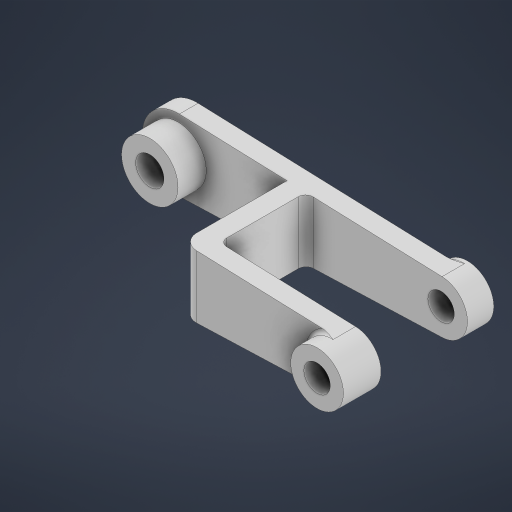
# Autodesk Inventor part: Part1
Saved by Autodesk Inventor 2023 (Build 270158000, 158)
## iProperties
Created: 2022-11-27
Part Number: Part1
Material: Generic
Document SubType Name: Modeling
Designer: iusti
Density: 1 g/cm^3
Appearance: Default
Author: iusti
Autodesk Inventor part; units mm, degrees
ref_plane "YZ Plane" through (0, 0, 0) normal (1, 0, 0) x (0, 1, 0)
ref_plane "XZ Plane" through (0, 0, 0) normal (0, 1, 0) x (-1, 0, 0)
sketch "Sketch1" plane through (0, 0, 0) normal (0, 0, 1) x (1, 0, 0)
  circle A0 centre (0, 0) radius 19
  circle A1 centre (140, 0) radius 14
  line L0 (0.678571, 18.987879) -> (140.5, 13.991069)
  line L1 (0.678571, -18.987879) -> (140.5, -13.991069)
  dimension "d0" = 38
  dimension "d1" = 28
  dimension "d2" = 140
  constraints: 4 end point, 4 point on circle, 4 tangent, 2 centre point, 1 coincident, 1 horizontal alignment
  measures "d0" diameter of A0
  measures "d1" diameter of A1
  measures "d2" distance of A1.centre point (0, 0)
extrude "Extrusion1" add sketch "Sketch1" along normal blind 10
ref_plane "Work Plane1" through (0, 0, 56) normal (0, 0, 1) x (1, 0, 0)
sketch "Sketch2" plane through (0, 0, 56) normal (0, 0, 1) x (1, 0, 0)
  line L0 (0.678571, -18.987879) -> (140.5, -13.991069) construction
  arc A0 (140.5, -13.991069) -> (140.5, 13.991069) centre (140, 0) ccw
  line L1 (140.5, 13.991069) -> (0.678571, 18.987879) construction
  arc A1 (0.678571, 18.987879) -> (0.678571, -18.987879) centre (0, 0) ccw construction
  line L2 (58, 16.939378) -> (58, -16.939378)
  line L3 (58, 16.939378) -> (140.5, 13.991069)
  line L4 (58, -16.939378) -> (140.5, -13.991069)
  arc A2 (140.5, -13.991069) -> (140.5, 13.991069) centre (140, 0) ccw
  dimension "d6" = 82
  constraints: 6 end point, 2 collinear, 2 point on circle, 2 point on line, 1 centre point, 1 coincident, 1 vertical
  measures "d6" distance from line of A0.centre L2
extrude "Extrusion2" add sketch "Sketch2" along normal blind 10
sketch "Sketch4" plane through (0, 0, 56) normal (0, 0, -1) x (-1, 0, 0)
  line L0 (-58, -16.939378) -> (-140.5, -13.991069)
  line L1 (-58, 16.939378) -> (-58, -16.939378)
  line L2 (-140.5, 13.991069) -> (-58, 16.939378)
  line L3 (-140.5, 13.991069) -> (-58, 16.939378)
  line L4 (-68, 16.582007) -> (-68, -16.582007)
  point P0 (0, 0)
  dimension "d10" = 10
  constraints: 2 end point, 2 point on line, 1 vertical
  measures "d10" distance between parallel lines of L1 L4
extrude "Extrusion3" add sketch "Sketch4" along normal up to next
fillet "Fillet1" radius 4 2 edges at (68, 0, 10) (68, 0, 56)
fillet "Fillet2" radius 8 1 edges at (58, 0, 66)
sketch "Sketch5" plane through (0, 0, 66) normal (0, 0, 1) x (1, 0, 0)
  arc A0 (140.5, -13.991069) -> (140.5, 13.991069) centre (140, 0) ccw
  line L0 (140.5, 13.991069) -> (72, 16.439059)
  circle A1 centre (140, 0) radius 14
  point P0 (0, 0)
  constraints: 1 coincident, 3 other
extrude "Extrusion4" add sketch "Sketch5" along normal blind 10
sketch "Sketch6" plane through (0, 0, 0) normal (0, 0, -1) x (-1, 0, 0)
  arc A0 (-140.5, 13.991069) -> (-140.5, -13.991069) centre (-140, 0) ccw
  line L0 (-140.5, 13.991069) -> (-72, 16.439059)
  circle A1 centre (-140, 0) radius 14
  point P0 (-140.5, -13.991069)
  constraints: 1 coincident, 3 other
extrude "Extrusion5" add sketch "Sketch6" along normal blind 4
sketch "Sketch7" plane through (140, 0, 76) normal (0, 0, 1) x (1, 0, 0)
  circle A0 centre (0, 0) radius 14 projected
  point P0 (-140, 0)
  constraints: 1 coincident
hole "Hole1" at (140, 0, 76) direction (0, 0, -1) diameter 14 end through all
sketch "Sketch8" plane through (0, 0, 10) normal (0, 0, 1) x (1, 0, 0)
  arc A0 (0.678571, 18.987879) -> (0.678571, -18.987879) centre (0, 0) ccw
  circle A1 centre (0, 0) radius 15
  dimension "d26" = 30
  constraints: 1 centre point, 1 coincident
  measures "d26" diameter of A1
extrude "Extrusion6" add sketch "Sketch8" along normal blind 15
sketch "Sketch10" plane through (0, 0, 25) normal (0, 0, 1) x (1, 0, 0)
  circle A0 centre (0, 0) radius 15 projected
  constraints: 1 coincident
hole "Hole2" at (0, 0, 25) direction (0, 0, -1) diameter 15 end through all
fillet "Fillet3" radius 2 2 edges at (126, 0, 0) (126, 0, 66)
body "Solid1"
